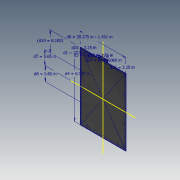
# Autodesk Inventor part: FLUGGER LOWER SIDE COVER
Saved by Autodesk Inventor 2020.3 (Build 243373000, 373)
## iProperties
RuleStatus: InUse
AfterDocSave0: file://Part Number Cleaner
Created: 2020-01-03
Material: ALUMINUM, 6061-T651
Vendor: HHMI: JRC - ID&F
Document SubType Name: Modeling
Designer: arnoldj
Density: 2.7 g/cm^3
Appearance: Anodized - Light Gray
DESIGN DEPARTMENT: HHMI: JRC - ID&F
ALTERED ITEM PART NUMBER: N/A
ALTERED ITEM VENDOR: N/A
ALTERED ITEM DESCRIPTION: N/A
Author: arnoldj
Revision Number: 0
Autodesk Inventor part; units mm, degrees
ref_plane "YZ Plane" through (0, 0, 0) normal (1, 0, 0) x (0, 1, 0)
ref_plane "XZ Plane" through (0, 0, 0) normal (0, 1, 0) x (-1, 0, 0)
ref_plane "XY Plane" through (0, 0, 0) normal (0, 0, 1) x (1, 0, 0)
sketch "Sketch1" plane through (0, 0, 0) normal (0, 0, 1) x (1, 0, 0)
  line L0 (0, 519.43) -> (0, -494.03) projected
  line L1 (-334.6907, 0) -> (334.6907, 0) projected
  line L2 (239.0648, -349.25) -> (-239.0648, -349.25)
  line L3 (-239.0648, -349.25) -> (-239.0648, 349.25)
  line L4 (-239.0648, 349.25) -> (239.0648, 349.25)
  line L5 (239.0648, 349.25) -> (239.0648, -349.25)
  line L6 (239.0648, -349.25) -> (-239.0648, 349.25) construction
  line L7 (-239.0648, -349.25) -> (239.0648, 349.25) construction
  line L8 (220.345, -330.5302) -> (-220.345, -330.5302) construction
  line L9 (-220.345, -330.5302) -> (-220.345, 330.5302) construction
  line L10 (-220.345, 330.5302) -> (220.345, 330.5302) construction
  line L11 (220.345, 330.5302) -> (220.345, -330.5302) construction
  line L12 (220.345, -330.5302) -> (-220.345, 330.5302) construction
  line L13 (-220.345, -330.5302) -> (220.345, 330.5302) construction
  line L14 (47.625, 374.65) -> (-47.625, 374.65)
  line L15 (-47.625, 374.65) -> (-47.625, 349.25)
  line L16 (-47.625, 349.25) -> (47.625, 349.25)
  line L17 (47.625, 349.25) -> (47.625, 374.65)
  line L18 (47.625, 374.65) -> (-47.625, 349.25) construction
  line L19 (-47.625, 374.65) -> (47.625, 349.25) construction
  point P0 (0, 0)
  point P1 (-156.5148, 330.5302)
  point P2 (0, 330.5302)
  point P3 (156.5148, 330.5302)
  point P4 (-156.5148, -330.5302)
  point P5 (0, -330.5302)
  point P6 (156.5148, -330.5302)
  point P7 (-220.345, 143.51)
  point P8 (-220.345, -143.51)
  point P9 (220.345, 143.51)
  point P10 (220.345, -117.0967)
  point P11 (-220.345, 0)
  point P12 (0, 361.95)
  point P13 (0, 361.6198)
  dimension "d0" = 478.1296
  dimension "d1" = 698.5
  dimension "d3" = 18.7198
  dimension "d4" = 18.7198
  dimension "d7" = 143.51
  dimension "d8" = 143.51
  dimension "d10" = 205.74
  dimension "d20" = 82.55
  dimension "d21" = 82.55
  dimension "d23" = 95.25
  dimension "d24" = 25.4
  dimension "d27" = 12.3698
  constraints: 36 end point, 11 point on line, 9 midpoint, 6 parallel, 4 coincident, 3 horizontal, 3 perpendicular, 2 vertical alignment, 1 horizontal alignment
  measures "d0" distance of L3.end L4.end
  measures "d1" distance of L2.end L3.end
  measures "d3" distance between parallel lines of L10 L4
  measures "d4" distance between parallel lines of L9 L3
  measures "d7" distance from line of L1 point (-220.345, 143.51)
  measures "d8" distance from line of point (-220.345, -143.51) L1
  measures "d10" distance from line of point (-220.345, 143.51) L4
  measures "d20" distance from line of point (-156.515, 330.53) L3
  measures "d21" distance from line of L5 point (156.515, 330.53)
  measures "d23" distance of L14.start L14.end
  measures "d24" distance of L14.end L15.end
  measures "d27" distance from line of L16 point (0, 361.62)
extrude "Extrusion1" add sketch "Sketch1" against normal blind 3.175
hole "Hole1" at (-156.5148, -330.5302, 0) at (156.5148, -330.5302, 0) at (220.345, 143.51, 0) at (220.345, -117.0967, 0) at (-220.345, 143.51, 0) at (-220.345, -143.51, 0) at (-220.345, 330.5302, 0) at (220.345, 330.5302, 0) at (0, 361.6198, 0) direction (0, 0, -1) diameter 8.255 end through all
fillet "Fillet1" radius 9.525 4 edges at (-239.0648, 349.25, -1.5875) (239.0648, 349.25, -1.5875) (239.0648, -349.25, -1.5875) (-239.0648, -349.25, -1.5875)
fillet "Fillet2" radius 3.175 4 edges at (47.625, 374.65, -1.5875) (47.625, 349.25, -1.5875) (-47.625, 374.65, -1.5875) (-47.625, 349.25, -1.5875)
body "Solid1"
